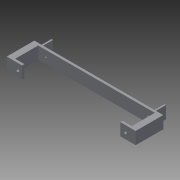
# Autodesk Inventor part: montowanie kostek ark do rozdzielnicy
Saved by Autodesk Inventor 2014 (Build 180170000, 170)
## iProperties
Created: 2018-03-25
Part Number: montowanie kostek ark do rozdzielnicy
Material: Generic
Document SubType Name: Modeling
Designer: HP820
Density: 1 g/cm^3
Appearance: Default
Author: HP820
Autodesk Inventor part; units mm, degrees
ref_plane "YZ Plane" through (0, 0, 0) normal (1, 0, 0) x (0, 1, 0)
ref_plane "XZ Plane" through (0, 0, 0) normal (0, 1, 0) x (-1, 0, 0)
ref_plane "XY Plane" through (0, 0, 0) normal (0, 0, 1) x (1, 0, 0)
sketch "Sketch1" plane through (0, 0, 0) normal (0, 1, 0) x (-1, 0, 0)
  line L0 (75, 8) -> (-75, 8)
  line L1 (-75, 8) -> (-75, -8)
  line L2 (-75, -8) -> (75, -8)
  line L3 (75, -8) -> (75, 8)
  line L4 (75, 8) -> (-75, -8) construction
  line L5 (-75, 8) -> (75, -8) construction
  line L6 (-75, 8) -> (-84, 8)
  line L7 (-84, 8) -> (-84, -8)
  line L8 (-84, -8) -> (-75, -8)
  line L9 (-75, -8) -> (-75, 8)
  line L10 (75, 8) -> (84, 8)
  line L11 (84, 8) -> (84, -8)
  line L12 (84, -8) -> (75, -8)
  line L13 (75, -8) -> (75, 8)
  point P0 (0, 0)
  dimension "d0" = 150
  dimension "d1" = 16
  dimension "d2" = 9
  dimension "d3" = 9
  constraints: 28 end point, 6 parallel, 3 horizontal, 3 perpendicular, 2 midpoint
  measures "d0" distance of L2.end L1.end
  measures "d1" distance between parallel lines of L0 L2
  measures "d2" distance of L8.end L7.end
  measures "d3" distance of L11.end L12.end
extrude "Extrusion1" add sketch "Sketch1" along normal blind 3
sketch "Sketch2" plane through (0, 3, 0) normal (0, 1, 0) x (1, 0, 0)
  line L0 (-70.5, 4.5) -> (70.5, 4.5)
  line L1 (70.5, 4.5) -> (70.5, -4.5)
  line L2 (70.5, -4.5) -> (-70.5, -4.5)
  line L3 (-70.5, -4.5) -> (-70.5, 4.5)
  line L4 (-70.5, 4.5) -> (70.5, -4.5) construction
  line L5 (70.5, 4.5) -> (-70.5, -4.5) construction
  circle A0 centre (-66.5, 0) radius 1.25
  circle A1 centre (-66.5, 0) radius 4
  circle A2 centre (66.5, 0) radius 1.25
  circle A3 centre (66.5, 0) radius 4
  point P0 (0, 0)
  dimension "d6" = 141
  dimension "d7" = 9
  dimension "d8" = 2.5
  dimension "d9" = 8
  dimension "d10" = 4
  dimension "d11" = 2.5
  dimension "d12" = 8
  dimension "d13" = 4
  constraints: 12 end point, 4 centre point, 2 coincident, 2 midpoint, 2 parallel, 1 horizontal, 1 perpendicular
  measures "d6" distance of L1.end L2.end
  measures "d7" distance of L0.end L1.end
  measures "d8" diameter of A0
  measures "d9" diameter of A1
  measures "d10" distance from line of L3 A1.centre
  measures "d11" diameter of A2
  measures "d12" diameter of A3
  measures "d13" distance from line of L1 A2.centre
extrude "Extrusion2" add sketch "Sketch2" along normal blind 3 contours A1 | A3
sketch "Sketch3" plane through (0, 3, 0) normal (0, 1, 0) x (1, 0, 0)
  circle A0 centre (-66.5, 0) radius 1.25 projected
  circle A1 centre (66.5, 0) radius 1.25 projected
  point P0 (0, 0)
extrude "Extrusion3" cut sketch "Sketch3" against normal blind 3
sketch "Sketch4" plane through (0, 3, 0) normal (0, 1, 0) x (1, 0, 0)
  line L0 (-62.5, 4.7822) -> (62.5, 4.7822)
  line L1 (62.5, 4.7822) -> (62.5, 3.2178)
  line L2 (62.5, 3.2178) -> (-62.5, 3.2178)
  line L3 (-62.5, 3.2178) -> (-62.5, 4.7822)
  line L4 (-62.5, 4.7822) -> (62.5, 3.2178) construction
  line L5 (62.5, 4.7822) -> (-62.5, 3.2178) construction
  point P0 (0, 0)
  point P1 (0, 4)
  constraints: 12 end point, 2 midpoint, 2 parallel, 1 horizontal, 1 perpendicular
extrude "Extrusion4" add sketch "Sketch4" along normal blind 3
sketch "Sketch5" plane through (0, 0, 0) normal (0, -1, 0) x (1, 0, 0)
  line L0 (84, -8) -> (-84, -8) projected
  line L1 (-84, 8) -> (-76, 8)
  line L2 (-76, 8) -> (-76, -8)
  line L3 (-76, -8) -> (-84, -8)
  line L4 (-84, -8) -> (-84, 8)
  line L5 (84, 8) -> (76, 8)
  line L6 (76, 8) -> (76, -8)
  line L7 (76, -8) -> (84, -8)
  line L8 (84, -8) -> (84, 8)
  point P0 (0, 0)
  dimension "d20" = 8
  dimension "d21" = 8
  constraints: 16 end point, 4 parallel, 2 horizontal, 2 perpendicular, 2 point on line
  measures "d20" distance of L2.end L3.end
  measures "d21" distance of L7.end L6.end
extrude "Extrusion5" add sketch "Sketch5" along normal blind 30
sketch "Sketch6" plane through (0, -30, 0) normal (0, -1, 0) x (1, 0, 0)
  line L0 (-84, 8) -> (-64, 8)
  line L1 (-64, 8) -> (-64, -8)
  line L2 (-64, -8) -> (-84, -8)
  line L3 (-84, -8) -> (-84, 8)
  point P0 (0, 0)
  dimension "d24" = 20
  constraints: 8 end point, 2 parallel, 1 horizontal, 1 perpendicular
  measures "d24" distance of L1.end L2.end
sketch "Sketch7" plane through (0, -30, 0) normal (0, -1, 0) x (1, 0, 0)
  line L0 (84, 8) -> (64, 8)
  line L1 (64, 8) -> (64, -8)
  line L2 (64, -8) -> (84, -8)
  line L3 (84, -8) -> (84, 8)
  point P0 (0, 0)
  dimension "d25" = 20
  constraints: 8 end point, 2 parallel, 1 horizontal, 1 perpendicular
  measures "d25" distance of L2.end L1.end
extrude "Extrusion6" add sketch "Sketch7" along normal blind 3
extrude "Extrusion7" add sketch "Sketch6" along normal blind 3
sketch "Sketch8" plane through (0, -33, 0) normal (0, -1, 0) x (1, 0, 0)
  line L0 (-84, -8) -> (-64, -8) projected
  line L1 (-76, -8) -> (-76, 8) projected
  line L2 (-64, 8) -> (-76, 8) projected
  line L3 (-64, -8) -> (-64, 8) projected
  line L4 (-76, -8) -> (-64, -8) projected
  circle A0 centre (-70, 0) radius 2.25
  point P0 (0, 0)
  dimension "d30" = 4.5
  constraints: 1 centre point
  measures "d30" diameter of A0
extrude "Extrusion8" cut sketch "Sketch8" against normal blind 3 contours A0
sketch "Sketch9" plane through (0, -33, 0) normal (0, -1, 0) x (1, 0, 0)
  line L0 (76, 8) -> (76, -8) projected
  line L1 (76, 8) -> (76, -8) projected
  line L2 (64, -8) -> (76, -8) projected
  line L3 (64, 8) -> (64, -8) projected
  line L4 (76, 8) -> (64, 8) projected
  circle A0 centre (70, 0) radius 2.25
  point P0 (0, 0)
  dimension "d33" = 4.5
  constraints: 1 centre point
  measures "d33" diameter of A0
extrude "Extrusion9" cut sketch "Sketch9" against normal blind 3 contours A0
sketch "Sketch11" plane through (0, 3, 0) normal (0, 1, 0) x (1, 0, 0)
  line L0 (-84, -8) -> (84, -8) projected
  line L1 (84, 8) -> (-84, 8) projected
  line L2 (-72.587, 8) -> (-74.587, 8)
  line L3 (-74.587, 8) -> (-74.587, -8)
  line L4 (-74.587, -8) -> (-72.587, -8)
  line L5 (-72.587, -8) -> (-72.587, 8)
  line L6 (-72.587, 8) -> (72.5136, 8)
  line L7 (72.5136, 8) -> (72.5136, 6.6306)
  line L8 (72.5136, 6.6306) -> (-72.587, 6.6306)
  line L9 (-72.587, 6.6306) -> (-72.587, 8)
  line L10 (72.5136, 8) -> (74.5136, 8)
  line L11 (74.5136, 8) -> (74.5136, -8)
  line L12 (74.5136, -8) -> (72.5136, -8)
  line L13 (72.5136, -8) -> (72.5136, 8)
  point P0 (0, 0)
  dimension "d38" = 2
  dimension "d39" = 2
  constraints: 24 end point, 6 parallel, 3 horizontal, 3 perpendicular, 3 point on line
  measures "d38" distance of L4.end L3.end
  measures "d39" distance of L11.end L12.end
extrude "Extrusion10" add sketch "Sketch11" along normal blind 13 contours L3 L1 L5 L0 | L13 L7 L1 L11 L0 | L5 L1 L7 L8
body "Solid1"
